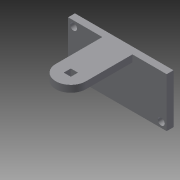
# Autodesk Inventor part: Autonomous - Ultrasonic to Servo
Saved by Autodesk Inventor 2015 (Build 190159000, 159)
## iProperties
Created: 2015-05-13
Part Number: Autonomous - Ultrasonic to Servo
Material: Generic
Document SubType Name: Modeling
Designer: 166189
Density: 1 g/cm^3
Appearance: Default
Author: 166189
Autodesk Inventor part; units mm, degrees
ref_plane "YZ Plane" through (0, 0, 0) normal (1, 0, 0) x (0, 1, 0)
ref_plane "XZ Plane" through (0, 0, 0) normal (0, 1, 0) x (-1, 0, 0)
ref_plane "XY Plane" through (0, 0, 0) normal (0, 0, 1) x (1, 0, 0)
sketch "Sketch1" plane through (0, 0, 0) normal (0, 1, 0) x (-1, 0, 0)
  circle A0 centre (0, 0) radius 6.985
  line L0 (6.985, 0) -> (6.985, -21.59)
  line L1 (6.985, -21.59) -> (-6.985, -21.59)
  line L2 (-6.985, -21.59) -> (-6.985, 0)
  line L3 (0, 0) -> (1.651, 0)
  line L4 (1.651, 0) -> (1.651, -1.651)
  line L5 (1.651, -1.651) -> (-1.651, -1.651)
  line L6 (-1.651, -1.651) -> (-1.651, 1.651)
  line L7 (-1.651, 1.651) -> (1.651, 1.651)
  line L8 (1.651, 1.651) -> (1.651, 0)
  dimension "d0" = 13.97
  dimension "d1" = 21.59
  dimension "d2" = 13.97
  dimension "d3" = 1.651
  dimension "d4" = 1.651
  dimension "d5" = 3.302
  dimension "d6" = 3.302
  dimension "d7" = 3.302
  constraints: 18 end point, 4 perpendicular, 2 point on circle, 1 centre point, 1 coincident, 1 collinear, 1 horizontal, 1 point on line, 1 tangent, 1 vertical
  measures "d0" diameter of A0
  measures "d1" distance of L0.start L0.end
  measures "d2" distance of L0.end L1.end
  measures "d3" distance of L3.start L3.end
  measures "d4" distance of L3.end L4.end
  measures "d5" distance of L4.end L5.end
  measures "d6" distance of L5.end L6.end
  measures "d7" distance of L6.end L7.end
extrude "Extrusion1" add sketch "Sketch1" along normal blind 3.175
sketch "Sketch2" plane through (6.985, 0, -21.59) normal (0, 0, -1) x (-1, 0, 0)
  line L0 (13.97, 3.175) -> (0, 3.175) projected
  line L1 (6.985, 3.175) -> (-15.875, 3.175)
  line L2 (-15.875, 3.175) -> (-15.875, -19.685)
  line L3 (-15.875, -19.685) -> (29.845, -19.685)
  line L4 (29.845, -19.685) -> (29.845, 3.175)
  line L5 (29.845, 3.175) -> (6.985, 3.175)
  point P0 (6.985, 0)
  dimension "d10" = 22.86
  dimension "d11" = 22.86
  dimension "d12" = 45.72
  constraints: 10 end point, 3 perpendicular, 2 collinear, 1 midpoint, 1 point on line
  measures "d10" distance of L1.start L1.end
  measures "d11" distance of L1.end L2.end
  measures "d12" distance of L2.end L3.end
extrude "Extrusion2" add sketch "Sketch2" along normal blind 3.175
sketch "Sketch3" plane through (6.985, 0, -24.765) normal (0, 0, -1) x (-1, 0, 0)
  line L0 (29.845, 3.175) -> (27.305, 3.175)
  line L1 (29.845, 3.175) -> (-15.875, 3.175) projected
  line L2 (27.305, 3.175) -> (27.305, 0.635)
  circle A0 centre (27.305, 0.635) radius 1.5875
  line L3 (-15.875, -19.685) -> (-13.335, -19.685)
  line L4 (-13.335, -19.685) -> (-13.335, -17.145)
  circle A1 centre (-13.335, -17.145) radius 1.5875
  point P0 (6.985, 0)
  dimension "d15" = 2.54
  dimension "d16" = 2.54
  dimension "d17" = 3.175
  dimension "d18" = 2.54
  dimension "d19" = 2.54
  dimension "d20" = 3.175
  constraints: 8 end point, 2 centre point, 2 coincident, 2 perpendicular, 1 horizontal, 1 point on line
  measures "d15" distance of L0.start L0.end
  measures "d16" distance of L0.end L2.end
  measures "d17" diameter of A0
  measures "d18" distance of L3.start L3.end
  measures "d19" distance of L3.end L4.end
  measures "d20" diameter of A1
extrude "Extrusion3" cut sketch "Sketch3" against normal blind 3.175
body "Solid1"
